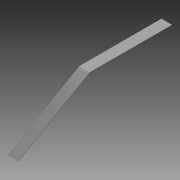
# Autodesk Inventor part: slats
Saved by Autodesk Inventor 2013 (Build 170138000, 138)
## iProperties
Created: 2012-12-18
Part Number: slats
Material: Steel, Carbon
Document SubType Name: Sheet Metal
Designer: istvan.burbank
Density: 7.87 g/cm^3
Sheet Metal Rule: Default
Flat Pattern Width: 7.62 cm
Flat Pattern Length: 118.231 cm
Flat Pattern Area: 900.921 cm^2
Sheet Metal Width: 3.000 in
Sheet Metal Length: 46.548 in
Sheet Metal Area: 139.643 in^2
Author: istvan.burbank
Autodesk Inventor part; units mm, degrees
ref_plane "YZ Plane" through (0, 0, 0) normal (1, 0, 0) x (0, 1, 0)
ref_plane "XZ Plane" through (0, 0, 0) normal (0, 1, 0) x (-1, 0, 0)
ref_plane "XY Plane" through (0, 0, 0) normal (0, 0, 1) x (1, 0, 0)
sketch "Sketch1" plane through (0, 0, 0) normal (0, 1, 0) x (-1, 0, 0)
  line L0 (0, 0) -> (76.2, 0)
  line L1 (76.2, 0) -> (76.2, 1828.8)
  line L2 (76.2, 1828.8) -> (0, 1828.8)
  line L3 (0, 1828.8) -> (0, 0)
  line L4 (0, 0) -> (25.4, 0)
  line L5 (0, 6.35) -> (0, 0)
  line L6 (0, 1828.8) -> (25.4, 1828.8)
  line L7 (0, 1822.45) -> (0, 1828.8)
  dimension "d0" = 76.2
  dimension "d1" = 1828.8
  constraints: 16 end point, 3 horizontal, 2 parallel, 1 perpendicular
  measures "d0" distance of L2.end L1.end
  measures "d1" distance of L1.end L0.end
extrude "Plate1" add sketch "Sketch1" along normal blind 3.175
sketch "Sketch2" plane through (0, 0, 0) normal (0, -1, 0) x (1, 0, 0)
  line L0 (0, 0) -> (-76.2, 0) projected
  line L1 (-76.2, 0) -> (-76.2, 1828.8) projected
  line L2 (-76.2, 1828.8) -> (0, 1828.8) projected
  line L3 (0, 1828.8) -> (0, 0) projected
  line L4 (-76.2, 914.4) -> (0, 914.4)
  point P0 (-25.4, 0)
  point P1 (-25.4, 1828.8)
  point P2 (0, 1822.45)
  point P3 (0, 6.35)
  dimension "d3" = -914.4
  dimension "d4" = -914.4
  constraints: 2 end point, 2 midpoint, 1 perpendicular
  measures "d3" distance between parallel lines of L0 L4
  measures "d4" distance between parallel lines of L2 L4
fold "Fold1" angle 30 bend radius 3.175 thickness 3.175 k factor 0.44 line from (-76.2, 0, 914.4) to (0, 0, 914.4) line at bend centre moving side (0, 0, 1) folds toward (0, -1, 0)
sketch "Sketch4" plane through (0, -457.0269, 1705.6476) normal (1, 0, 0) x (0, 0.5, -0.8660254)
  line L0 (913.2031, 3.175) -> (0, 3.175) projected
  line L1 (0, 0) -> (0, 3.175) projected
  line L2 (0, 0) -> (913.2031, 0) projected
  line L3 (916.3781, 2.3243) -> (914.7906, -0.4254) projected
  line L4 (914.7906, -0.4254) -> (1705.6476, -457.0269) projected
  line L5 (1705.6476, -457.0269) -> (1707.2351, -454.2773) projected
  line L6 (1707.2351, -454.2773) -> (916.3781, 2.3243) projected
  line L7 (323.2442, 0) -> (1425.7099, -295.4048)
  line L8 (1425.7099, -295.4048) -> (1427.2974, -292.6552)
  line L9 (323.2442, 0) -> (323.2442, 3.175)
  dimension "d22" = 589.9589
  dimension "d23" = 589.9589
  dimension "d34" = 1143
  constraints: 6 end point, 4 point on line, 2 perpendicular
  measures "d22" distance of L3.end L7.end
  measures "d23" distance of L7.start L2.end
  measures "d34" distance of L8.end L9.end
extrude "Extrusion2" cut sketch "Sketch4" against normal through all contours L9 L2 L1 L0 | L6 L5 L4 L8
ref_plane "Work Plane1" through (-19.05, 0, 323.2442) normal (0, -0.9659258, -0.258819) x (1, 0, 0)
equation "\"d3\" = d4"
equation "\"d5\" = BendReliefWidth"
equation "\"d6\" = BendReliefDepth"
equation "\"d7\" = MinimumRemnant"
equation "\"d8\" = BendRadius"
equation "\"d10\" = BendRadius"
equation "\"d22\" = d23"
equation "\"BendRadius\" = Thickness"
equation "\"BendReliefWidth\" = Thickness"
equation "\"BendReliefDepth\" = 0.5 * Thickness"
equation "\"CornerReliefSize\" = 4 * Thickness"
equation "\"MinimumRemnant\" = 2 * Thickness"
equation "\"TransitionRadius\" = BendRadius"
equation "\"JacobiRadiusSize\" = BendRadius"
equation "\"GapSize\" = Thickness"
equation "\"d2\" = BendRadius"
equation "\"Thickness\" = 3.175"
body "Solid1"
